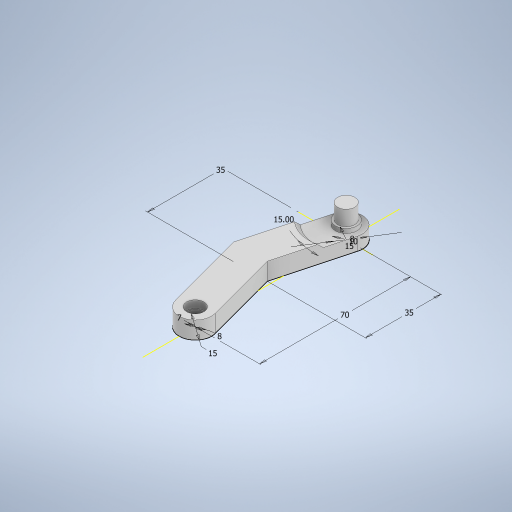
# Autodesk Inventor part: side arm
Saved by Autodesk Inventor 2024 (Build 280153000, 153)
## iProperties
Created: 2024-04-11
Part Number: side arm
Material: Generic
Document SubType Name: Modeling
Designer: compu
Density: 1 g/cm^3
Appearance: Default
Author: compu
Autodesk Inventor part; units mm, degrees
ref_plane "YZ Plane" through (0, 0, 0) normal (1, 0, 0) x (0, 1, 0)
ref_plane "XZ Plane" through (0, 0, 0) normal (0, 1, 0) x (-1, 0, 0)
ref_plane "XY Plane" through (0, 0, 0) normal (0, 0, 1) x (1, 0, 0)
sketch "Sketch3" plane through (0, 0, 0) normal (0, 1, 0) x (-1, 0, 0)
  circle A0 centre (0, 0) radius 4
  circle A1 centre (0, 0) radius 5
  circle A2 centre (0, 0) radius 7.5
  line L0 (0, -24.5) -> (0, 94.5) projected
  line L1 (22.0714, 0) -> (-12.4286, 0) projected
  circle A3 centre (0, 70) radius 4
  line L2 (7.2444, -1.9411) -> (17.1428, 35)
  line L3 (17.1428, 35) -> (7.2444, 71.9411)
  circle A4 centre (0, 70) radius 7.5
  line L4 (-7.2444, 1.9411) -> (1.6137, 35)
  line L5 (1.6137, 35) -> (-7.2444, 68.0589)
  circle A5 centre (0, 70) radius 3.5
  dimension "d15" = 8
  dimension "d16" = 10
  dimension "d17" = 15
  dimension "d18" = 8
  dimension "d19" = 70
  dimension "d20" = 15
  dimension "d21" = 35
  dimension "d24" = 15
  dimension "d25" = 35
  dimension "d43" = 7
  constraints: 8 end point, 6 centre point, 5 coincident, 4 point on circle, 4 tangent, 1 parallel, 1 point on line
  measures "d15" diameter of A0
  measures "d16" diameter of A1
  measures "d17" diameter of A2
  measures "d18" diameter of A3
  measures "d19" distance of point (0, 0) A3.centre
  measures "d20" diameter of A4
  measures "d21" distance from line of L1 L2.end
  measures "d24" angle of L0 L2
  measures "d25" distance from line of L1 L4.end
  measures "d43" diameter of A5
extrude "Extrusion4" add sketch "Sketch3" along normal blind 8 contours L1 L2 A2 | A2 L0 L4 L5 A4 L3 L2 L1 | A2 L4 L0 | L5 A4 L0
extrude "Extrusion5" add sketch "Sketch3" along normal blind 8 contours L1 A2 L0 A1 | A1 L0 A2 L1 | A1 L1 A2 L0 | L0 A2 L1 A1
sketch "Sketch4" plane through (0, 8, 0) normal (0, 1, 0) x (1, 0, 0)
  circle A0 centre (0, 0) radius 15
  circle A1 centre (0, 0) radius 13.25
  dimension "d30" = 30
  dimension "d31" = 26.5
  constraints: 2 centre point, 2 coincident
  measures "d30" diameter of A0
  measures "d31" diameter of A1
extrude "Extrusion6" cut sketch "Sketch4" against normal blind 2 contours A0 | A1
extrude "Extrusion7" add sketch "Sketch3" along normal blind 15 contours L1 L0 A0 | A0 L0 L1 | L0 L1 A0 | A0 L1 L0
extrude "Extrusion8" add sketch "Sketch3" along normal blind 8 contours L1 A1 L0 A0 | A0 L0 A1 L1 | A0 L1 A1 L0 | L0 A1 L1 A0
chamfer "Chamfer1" distance 2 angle 45 1 edges at (-3.8823, 8, 14.4889)
extrude "Extrusion9" add sketch "Sketch3" along normal blind 8 contours A4 L0 A3 | A4 L0 A3
extrude "Extrusion10" add sketch "Sketch3" along normal blind 4.5 contours A3 L0 A5 | L0 A5 A3
body "Solid2"
